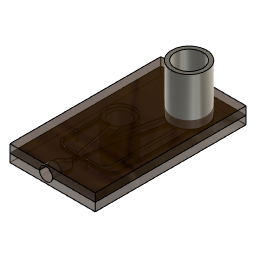
Valve_PEEP v5 (Autodesk Fusion 360 design; units mm, degrees)
Autodesk Fusion 360 part; units mm, degrees
sketch "Channels" plane through (0, 0, 0) normal (0, 0, 1) x (1, 0, 0)
  line L0 (0, 0) -> (46.5, 0)
  line L1 (46.5, 0) -> (46.5, 83) construction
  line L2 (46.5, 83) -> (0, 83) construction
  line L3 (0, 83) -> (0, 0)
  line L4 (27.5, -7) -> (27.5, 90) construction
  line L5 (10.6, 83) -> (10.6, 31.27) construction
  line L6 (46.5, 25.27) -> (16.6, 25.27) construction
  arc A0 (10.6, 31.27) -> (16.6, 25.27) centre (16.6, 31.27) ccw construction
  arc A1 (9.83, 31.27) -> (16.6, 24.5) centre (16.6, 31.27) ccw
  arc A2 (11.37, 31.27) -> (16.6, 26.04) centre (16.6, 31.27) ccw
  line L7 (27.5, 48.6) -> (34.6997, 83.1362)
  line L8 (27.5, 48.6) -> (46.5, 48.6) construction
  line L9 (27.5, 48.6) -> (25.0136, 60.5271)
  line L10 (25.8031, 26.04) -> (19.3855, 56.8243)
  line L11 (27.5, 17.9) -> (28.8759, 24.5) construction
  line L12 (29.1969, 26.04) -> (33.9, 48.6) construction
  line L13 (28.35, 24.5) -> (28.35, 21)
  line L14 (26.65, 24.5) -> (26.65, 21)
  arc A3 (28.35, 21) -> (30.6235, 17.0635) centre (32.8947, 21) ccw
  arc A4 (24.3765, 17.0635) -> (26.65, 21) centre (22.1053, 21) ccw
  line L15 (40.5, 26.04) -> (29.1969, 26.04)
  line L16 (25.8031, 26.04) -> (16.6, 26.04)
  line L17 (46.5, 24.5) -> (28.35, 24.5)
  line L18 (26.65, 24.5) -> (16.6, 24.5)
  line L19 (11.37, 57.9106) -> (11.37, 31.27)
  line L20 (9.83, 59.002) -> (9.83, 31.27)
  arc A5 (25.0136, 60.5271) -> (9.83, 59.002) centre (16.69, 67.05) ccw
  arc A6 (11.37, 57.9106) -> (19.3855, 56.8243) centre (16.69, 67.05) ccw
  circle A7 centre (16.69, 67.05) radius 7.5 construction
  line L21 (32.5, 0) -> (32.5, 7.9)
  line L22 (22.5, 0) -> (22.5, 7.9)
  arc A8 (24.3766, 17.0636) -> (22.5, 7.9) centre (27.5, 11.65) ccw
  arc A9 (22.5, 7.9) -> (27.5, 5.4) centre (27.5, 11.65) ccw construction
  arc A10 (27.5, 5.4) -> (32.5, 7.9) centre (27.5, 11.65) ccw construction
  arc A11 (32.5, 7.9) -> (30.6235, 17.0635) centre (27.5, 11.65) ccw
  line L23 (29.1969, 26.04) -> (40.5131, 80.3225)
  line L24 (40.5131, 80.3225) -> (44.213, 98.0704) construction
  line L25 (34.6997, 83.1362) -> (34.6713, 83) construction
  arc A12 (30.6235, 17.0635) -> (27.5, 17.9) centre (27.5, 11.65) ccw construction
  arc A13 (24.3765, 17.0635) -> (30.6235, 17.0635) centre (27.5, 11.65) ccw
  arc A14 (27.5, 17.9) -> (24.3765, 17.0635) centre (27.5, 11.65) ccw construction
  circle A15 centre (16.69, 67.05) radius 11.125 construction
  circle A16 centre (43.2274, 93.3425) radius 13.3
  line L26 (52.5, 83.8079) -> (52.5, 31.27) construction
  arc A17 (46.5, 25.27) -> (52.5, 31.27) centre (46.5, 31.27) ccw construction
  line L27 (53.27, 31.27) -> (53.27, 84.6226)
  arc A18 (46.5, 24.5) -> (53.27, 31.27) centre (46.5, 31.27) ccw
  line L28 (0, 83) -> (0, 115)
  line L29 (0, 115) -> (65, 115)
  line L30 (65, 115) -> (65, 0)
  line L31 (65, 0) -> (46.5, 0)
  line L32 (46.5, 80.4514) -> (46.5, 32.04)
  arc A19 (40.5, 26.04) -> (46.5, 32.04) centre (40.5, 32.04) ccw
  dimension "d1" = 83
  dimension "d2" = 46.5
  dimension "d6" = 6
  dimension "d7" = 10.6
  dimension "d8" = 25.27
  dimension "d11" = 12.5
  dimension "d12" = 12.85
  dimension "d13" = 34.4
  dimension "d14" = 12.6
  dimension "d16" = 3.3939
  dimension "d17" = 0.85
  dimension "d20" = 21.15
  dimension "d21" = 16.69
  dimension "d22" = 15.95
  dimension "d23" = 0.77
  dimension "d24" = 0.77
  dimension "d25" = 11.776
  dimension "d26" = 15
  dimension "d27" = 5
  dimension "d34" = 1.54
  dimension "d35" = 1.7
  dimension "d36" = 6.2653
  dimension "d38" = 3.5
  dimension "d65" = 22.25
  dimension "d78" = 26.6
  dimension "d81" = 27.5
  dimension "d82" = 6
  dimension "d84" = 0.77
  dimension "d87" = 115
  dimension "d94" = 6
  constraint horizontal L0
  constraint vertical L1
  constraint horizontal L2
  constraint vertical L3
  constraint coincident L0.start L3.end
  constraint perpendicular L2 L4
  constraint perpendicular L2 L5
  constraint coincident L1 L6.start
  constraint coincident L5 L5.start
  constraint coincident L2 L5.start
  constraint tangent L6 A0
  constraint tangent L5 A0
  constraint coincident L4 A8.centre
  constraint coincident L4 L7.start
  constraint coincident L2 L25.end
  constraint coincident L4 L11.start
  constraint perpendicular L4 L8
  constraint coincident L12.end L8
  constraint parallel L11 L23
  constraint parallel L7 L23
  constraint symmetric L4 L7.start L8.start
  constraint coincident L11.end L17
  constraint collinear L11 L12
  constraint coincident L10.start L15
  constraint perpendicular L13 L17
  constraint symmetric L4 L13.start L14.start
  constraint tangent L13 A3
  constraint coincident A3.end A8
  constraint symmetric L4 A3.end A4.start
  constraint symmetric L4 L13.end L14.end
  constraint symmetric L4 A3 A4
  constraint parallel L6 L15
  constraint concentric A0 A2
  constraint tangent A2 L15
  constraint collinear L15 L16
  constraint parallel L6 L17
  constraint concentric A0 A1
  constraint tangent A1 L17
  constraint collinear L17 L18
  constraint coincident A3 A11.end
  constraint coincident A4 A8.start
  constraint coincident L19.start A5
  constraint tangent A1 L20
  constraint concentric A5 A6
  constraint concentric A6 A7
  constraint coincident L1 L8.end
  constraint coincident L0 L21.start
  constraint coincident L21.end A8
  constraint perpendicular L0 L21
  constraint symmetric L4 L21.start L22.start
  constraint symmetric L4 L21.end L22.end
  constraint coincident L4 A9.end
  constraint concentric A8 A10
  constraint concentric A8 A9
  constraint concentric A10 A12
  constraint concentric A10 A11
  constraint parallel L9 L10
  constraint parallel L23 L25
  constraint tangent A3 A11
  constraint concentric A12 A13
  constraint concentric A12 A14
  constraint concentric A5 A15
  constraint collinear L23 L24
  constraint coincident L24 A16.centre
  constraint coincident A16 L26.start
  constraint parallel L1 L26
  constraint tangent L6 A17
  constraint tangent L26 A17
  constraint coincident A16 L27.end
  constraint parallel L26 L27
  constraint coincident L1 L17.start
  constraint coincident L23.end A16
  constraint tangent L27 A18
  constraint perpendicular L2 L28
  constraint perpendicular L3 L29
  constraint perpendicular L29 L30
  constraint perpendicular L1 L31
  constraint coincident A16 L32.start
  constraint coincident L1 L32.start
  constraint tangent L15 A19
  constraint tangent L32 A19
  constraint coincident L7.end A16
  measures "d1" distance of L0.start L2.end
  measures "d2" distance of L0.start L0.end
  measures "d6" radius of A0
  measures "d7" distance of L3 L5
  measures "d8" distance of L0 L6
  measures "d11" diameter of A8
  measures "d12" distance of A8.centre L17
  measures "d13" distance of L2 L7.start
  measures "d14" distance of L1 L12.end
  measures "d16" distance of L12.start L10.start
  measures "d17" distance of L4 L13
  measures "d20" diameter of A5
  measures "d21" distance of L3 A5.centre
  measures "d22" distance of L2 A5.centre
  measures "d23" distance of L5 L19
  measures "d24" distance of L5 L20
  measures "d25" angle of L4 L7
  measures "d26" diameter of A7
  measures "d27" distance of L4 L21
  measures "d34" distance of L19 L20
  measures "d35" distance of L13 L14
  measures "d36" distance of L7 L23
  measures "d38" distance of L14.start L14.end
  measures "d65" diameter of A15
  measures "d78" diameter of A16
  measures "d81" horizontal distance of A8.centre L0.start
  measures "d82" radius of A17
  measures "d84" distance of L26 L27
  measures "d87" distance of L0.start L29
  measures "d94" radius of A19
sketch "Set screws" plane through (0, 0, 0) normal (0, 0, 1) x (1, 0, 0)
  line L0 (46.5, 25.27) -> (16.6, 25.27) construction
  line L1 (27.5, -7) -> (27.5, 90) construction
  arc A0 (10.6, 31.27) -> (16.6, 25.27) centre (16.6, 31.27) ccw construction
  line L2 (10.6, 83) -> (10.6, 31.27) construction
  circle A1 centre (33, 25.27) radius 1.25
  circle A2 centre (10.6, 40.27) radius 1.25
  dimension "d61" = 2.5
  dimension "d62" = 2.5
  dimension "d63" = 5.5
  dimension "d64" = 15
  constraint coincident L0 A1.centre
  constraint coincident L2 A2.centre
  measures "d61" diameter of A1
  measures "d62" diameter of A2
  measures "d63" distance of L1 A1.centre
  measures "d64" distance of L0 A2.centre
extrude "Extrude1" add sketch "Channels" along normal blind 6.25 and the other way blind 6.25 contours L0 L3 A1 L7 L9 L13 L14 A3 A4 L17 L18 L20 A5 L21 L22 A8 A11 A13 A16 L27 A18 L28 L29 L30 L31 | L0 L21 L22 A13 | A1 L7 L9 L13 L14 A3 A4 L15 L17 L18 L20 A5 A8 A11 L23 A13 A16 L27 A18 L32 A19 | A16 | L15 L23 A16 L32 A19 | A2 L10 L16 L19 A6 makes body 1
extrude "Extrude2" cut sketch "Channels" against normal blind 2.25 contours A1 L7 L9 L13 L14 A3 A4 L15 L17 L18 L20 A5 A8 A11 L23 A13 A16 L27 A18 L32 A19 | A16 bodies 1
extrude "Extrude9" cut sketch "Set screws" against normal through all bodies 1
ref_plane "WorkPlane1" through (0, 67.05, 0) normal (0, 1, 0) x (0, 0, 1)
sketch "Outlet" plane through (0, 67.05, 0) normal (0, 1, 0) x (1, 0, 0)
  line L0 (27.265, 0) -> (27.265, 2.25)
  line L1 (27.265, 2.25) -> (27.815, 2.25)
  line L2 (27.815, 2.25) -> (27.815, 20)
  line L3 (27.815, 20) -> (27.54, 28.03)
  line L4 (24.19, 0) -> (24.19, 28.03)
  line L5 (24.19, 28.03) -> (27.54, 28.03)
  line L6 (27.265, 2.25) -> (24.19, 2.25)
  line L7 (27.265, 0) -> (24.19, 0)
  line L8 (16.69, 0) -> (16.69, 56) construction
  line L9 (24.19, 0) -> (16.69, 0)
  line L10 (24.19, 28.03) -> (16.69, 28)
  line L11 (16.69, 0) -> (16.69, 28)
  point P0 (9.19, 0)
  point P1 (24.19, 0)
  point P2 (27.265, 0)
  point P3 (6.115, 0)
  point P4 (5.565, 0)
  point P5 (27.815, 0)
  point P6 (16.69, 0)
  dimension "d67" = 17.75
  dimension "d68" = 25.78
  dimension "d69" = 7.5
  dimension "d70" = 11.125
  dimension "d71" = 2.25
  dimension "d74" = 10.85
  constraint coincident P2 L0.start
  constraint vertical L0
  constraint perpendicular L0 L1
  constraint perpendicular L1 L2
  constraint coincident P1 L4.start
  constraint vertical L4
  constraint horizontal L5
  constraint coincident L4 L6.end
  constraint perpendicular L4 L6
  constraint coincident P5 L2
  constraint coincident P6 L8.start
  constraint vertical L8
  constraint midpoint L8 L10.end
  measures "d67" distance of L1.end L2.end
  measures "d68" distance of L4.end L6.end
  measures "d69" distance of P6 L4
  measures "d70" distance of P5 L8.start
  measures "d71" distance of P2 L6
  measures "d74" horizontal distance of P6 L3.end
revolve "Revolve1" cut sketch "Outlet" angle 360 about axis through (16.69, 67.05, 0) along (0, 0, -1) bodies 1
revolve "Revolve2" add sketch "Outlet" angle 360 about axis through (16.69, 67.05, 0) along (0, 0, -1) separate body contours L1 L2 L3 L4 L5 L6 makes body 2
sketch "Inlet" plane through (0, 0, 0) normal (0, -1, 0) x (1, 0, 0)
  line L0 (65, 6.25) -> (0, 6.25)
  line L1 (0, 6.25) -> (0, -6.25)
  line L2 (0, -6.25) -> (65, -6.25)
  circle A0 centre (27.5, 0) radius 5
  line L3 (65, -6.25) -> (65, 6.25)
  point P0 (27.5, 0)
  point P1 (22.5, 0)
  constraint coincident P0 A0.centre
  constraint coincident P1 A0
extrude "Extrude5" cut sketch "Inlet" against normal blind 6.7 contours A0 bodies 1
split "Split1" by plane through (0, 0, 0) normal (0, 0, 1) bodies 1 makes body 3 at (21.6667, 76.6667, 6.25)
sketch "Sketch7" plane through (0, 0, 6.25) normal (0, 0, 1) x (-1, 0, 0)
  line L0 (0, -115) -> (0, 0)
  line L1 (0, 0) -> (-65, 0)
  line L2 (-65, 0) -> (-65, -115)
  line L3 (-65, -115) -> (0, -115)
  circle A0 centre (-43.2274, -93.3425) radius 13.3 construction
  circle A1 centre (-43.2274, -93.3425) radius 10.46
  circle A2 centre (-43.2274, -93.3425) radius 13.3
  dimension "d85" = 20.92
  dimension "d95" = 26.6
  constraint concentric A0 A1
  constraint concentric A1 A2
  measures "d85" diameter of A1
  measures "d95" diameter of A2
extrude "Extrude10" cut sketch "Sketch7" against normal up to surface (6.25 mm away) contours A1 | A2 bodies 1
extrude "Extrude11" add sketch "Sketch7" along normal blind 30 and the other way up to surface (6.25 mm away) separate body contours A2 makes body 4
thread "Thread1" "ISO Metric profile 3.0 M3x0.5 6H" major diameter 3.086 minor diameter 2.529 pitch 0.5 angle 60 resizes the face on face at (9.3533, 40.1787, -4.1667) on face at (32.1438, 24.3593, -4.1667) on bodies 1
equation "d12 = ( 12.5 / 2 ) * 1 mm + 6.60 mm"
equation "d74 = ( 21.7 / 2 ) * 1 mm"
named bodies: "Top half", "Output adapter", "Bottom half", "PEEP reservoir"
